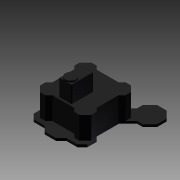
# Autodesk Inventor part: Base
Saved by Autodesk Inventor 2012 (Build 160160000, 160)
## iProperties
Created: 2013-03-08
Part Number: Base
Material: Default
Document SubType Name: Modeling
Designer: Andrew
Density: 1 g/cm^3
Author: Andrew
Autodesk Inventor part; units mm, degrees
ref_plane "YZ Plane" through (0, 0, 0) normal (1, 0, 0) x (0, 1, 0)
ref_plane "XZ Plane" through (0, 0, 0) normal (0, 1, 0) x (-1, 0, 0)
ref_plane "XY Plane" through (0, 0, 0) normal (0, 0, 1) x (1, 0, 0)
sketch "Sketch1" plane through (0, 0, 0) normal (0, 0, 1) x (1, 0, 0)
  line L0 (87.39809, 90.638849) -> (76.791489, 101.245451)
  line L1 (110.603697, 90.638591) -> (87.39809, 90.638849)
  line L2 (121.210063, 101.244956) -> (110.603697, 90.638591)
  line L3 (143.419374, 101.244709) -> (121.210063, 101.244956)
  line L4 (153.419263, 111.244598) -> (143.419374, 101.244709)
  line L5 (153.419473, 130.081843) -> (153.419263, 111.244598)
  line L6 (144.001258, 139.500058) -> (153.419473, 130.081843)
  line L7 (144.001258, 184.500058) -> (144.001258, 139.500058)
  line L8 (162.838724, 203.336883) -> (144.001258, 184.500058)
  line L9 (174.479779, 203.336684) -> (162.838724, 203.336883)
  line L10 (188.623093, 217.476415) -> (174.479779, 203.336684)
  line L11 (188.623904, 237.476415) -> (188.623093, 217.476415)
  line L12 (174.481567, 251.622561) -> (188.623904, 237.476415)
  line L13 (154.481567, 251.622902) -> (174.481567, 251.622561)
  line L14 (140.33919, 237.481007) -> (154.481567, 251.622902)
  line L15 (140.338992, 225.83779) -> (140.33919, 237.481007)
  line L16 (121.502223, 207.001664) -> (140.338992, 225.83779)
  line L17 (76.502223, 207.001664) -> (121.502223, 207.001664)
  line L18 (57.665842, 225.839164) -> (76.502223, 207.001664)
  line L19 (57.66604, 237.480627) -> (57.665842, 225.839164)
  line L20 (43.524145, 251.623004) -> (57.66604, 237.480627)
  line L21 (23.524145, 251.623344) -> (43.524145, 251.623004)
  line L22 (9.381769, 237.48145) -> (23.524145, 251.623344)
  line L23 (9.380958, 217.48145) -> (9.381769, 237.48145)
  line L24 (23.52252, 203.338741) -> (9.380958, 217.48145)
  line L25 (35.165328, 203.338269) -> (23.52252, 203.338741)
  line L26 (54.001421, 184.501058) -> (35.165328, 203.338269)
  line L27 (54.001421, 139.501058) -> (54.001421, 184.501058)
  line L28 (44.582671, 130.082867) -> (54.001421, 139.501058)
  line L29 (44.582461, 111.245809) -> (44.582671, 130.082867)
  line L30 (54.582226, 101.245698) -> (44.582461, 111.245809)
  line L31 (76.791489, 101.245451) -> (54.582226, 101.245698)
  circle A0 centre (99, 132) radius 5.5
  arc A1 (130.06, 142) -> (135.06, 142) centre (132.56, 142) ccw
  line L32 (130.06, 142) -> (130.06, 182)
  line L33 (135.06, 182) -> (135.06, 142)
  arc A2 (62.940969, 142) -> (67.940969, 142) centre (65.440969, 142) ccw
  arc A3 (67.940969, 182) -> (62.940969, 182) centre (65.440969, 182) ccw
  line L34 (67.940969, 182) -> (67.940969, 142)
  line L35 (138.997508, 214.221497) -> (150.997508, 202.221497)
  line L36 (128.721743, 214.221497) -> (138.997508, 214.221497)
  line L37 (121.5, 207) -> (128.721743, 214.221497)
  line L38 (76.5, 207) -> (121.5, 207)
  line L39 (69.278592, 214.221497) -> (76.5, 207)
  line L40 (59.002492, 214.221497) -> (69.278592, 214.221497)
  line L41 (47.002492, 202.221497) -> (59.002492, 214.221497)
  line L42 (47.002492, 191.497594) -> (47.002492, 202.221497)
  line L43 (54, 184.5) -> (47.002492, 191.497594)
  line L44 (54, 139.5) -> (54, 184.5)
  line L45 (47.002492, 132.502579) -> (54, 139.5)
  line L46 (47.002492, 121.778503) -> (47.002492, 132.502579)
  line L47 (59.002492, 109.778503) -> (47.002492, 121.778503)
  line L48 (69.278414, 109.778503) -> (59.002492, 109.778503)
  line L49 (76.5, 117) -> (69.278414, 109.778503)
  line L50 (121.5, 117) -> (76.5, 117)
  line L51 (128.721408, 109.778503) -> (121.5, 117)
  line L52 (138.997508, 109.778503) -> (128.721408, 109.778503)
  line L53 (150.997508, 121.778503) -> (138.997508, 109.778503)
  line L54 (150.997508, 132.502406) -> (150.997508, 121.778503)
  line L55 (144, 139.5) -> (150.997508, 132.502406)
  line L56 (144, 184.5) -> (144, 139.5)
  line L57 (150.997508, 191.497269) -> (144, 184.5)
  line L58 (150.997508, 202.221497) -> (150.997508, 191.497269)
  arc A4 (99.74629, 120.775345) -> (99.246799, 120.752769) centre (99, 131.75) ccw
  line L59 (111.585786, 133.75) -> (111, 133.75)
  line L60 (111.585786, 133.75) -> (111.585786, 135.25)
  line L61 (111.585786, 135.25) -> (113.5, 135.25)
  line L62 (113.5, 135.45) -> (113.5, 135.25)
  line L63 (113.5, 135.45) -> (113.917157, 135.45)
  line L64 (113.917157, 135.45) -> (113.917157, 141.55)
  line L65 (110.05, 169.167157) -> (103.95, 169.167157)
  line L66 (103.95, 169.167157) -> (103.95, 166.667157)
  line L67 (103.95, 166.667157) -> (94.05, 166.667157)
  line L68 (94.05, 166.667157) -> (94.05, 169.167157)
  line L69 (87.95, 169.167157) -> (87.95, 168.75)
  line L70 (87.95, 168.75) -> (87.5, 168.75)
  line L71 (86.414214, 135.25) -> (84.5, 135.25)
  line L72 (86.414214, 135.25) -> (86.414214, 133.75)
  line L73 (86.414214, 133.75) -> (87, 133.75)
  line L74 (87, 133.75) -> (87, 125.5)
  line L75 (87, 125.5) -> (89, 125.5)
  line L76 (109, 125.5) -> (111, 125.5)
  line L77 (111, 125.5) -> (111, 133.75)
  line L78 (85, 136.25) -> (86, 136.25)
  line L79 (86, 136.25) -> (86, 137.354356)
  line L80 (104.686492, 167.25) -> (104.686492, 168.25)
  line L81 (104.686492, 168.25) -> (105.854356, 168.25)
  line L82 (105.854356, 167.25) -> (104.686492, 167.25)
  circle A5 centre (99, 131.75) radius 11
  point P0 (0, 0)
  point P1 (0, 0)
  constraints: 64 end point, 1 centre point, 1 coincident, 1 concentric
extrude "Extrusion1" add sketch "Sketch1" along normal blind 5 contours L0 L31 L30 L29 L28 L46 L47 L48 L49 L50 L51 L52 L53 L54 L6 L5 L4 L3 L2 L1 | L28 L27 L26 L42 L41 L40 L39 L17 L16 L36 L35 L58 L8 L7 L6 L54 L53 L52 L51 L50 L49 L48 L47 L46 | L26 L25 L24 L23 L22 L21 L20 L19 L18 L39 L40 L41 L42 | L58 L35 L36 L16 L15 L14 L13 L12 L11 L10 L9 L8 | A0 | A5 A4
extrude "Extrusion2" add sketch "Sketch1" along normal blind 50.4 contours L28 L27 L26 L42 L41 L40 L39 L17 L16 L36 L35 L58 L8 L7 L6 L54 L53 L52 L51 L50 L49 L48 L47 L46 | A0 | A5 A4
extrude "Extrusion3" add sketch "Sketch1" along normal blind 87.4 contours A0 | A5 A4
sketch "Sketch2" plane through (0, 0, 50.4) normal (0, 0, 1) x (1, 0, 0)
  circle A0 centre (99, 131.75) radius 11 projected
  line L0 (144, 184.5) -> (144, 139.5) projected
  line L1 (99, 120.75) -> (112, 120.75)
  line L2 (112, 120.75) -> (112, 165.75)
  line L3 (112, 165.75) -> (86, 165.75)
  line L4 (86, 165.75) -> (86, 120.75)
  line L5 (86, 120.75) -> (99, 120.75)
  point P0 (0, 0)
  dimension "d6" = 13
  dimension "d7" = 45
  dimension "d8" = 26
  constraints: 10 end point, 2 parallel, 2 perpendicular, 1 horizontal, 1 vertical alignment, 1 other
  measures "d6" distance of L1.start L1.end
  measures "d7" distance of L1.end L2.end
  measures "d8" distance of L2.end L3.end
extrude "Extrusion4" add sketch "Sketch2" along normal blind 34
fillet "Fillet1" radius 2 7 edges at (112, 165.75, 67.4) (112, 143.25, 84.4) (112, 120.75, 67.4) (86, 120.75, 67.4) (86, 143.25, 84.4) (99, 165.75, 84.4) (86, 165.75, 67.4)
body "Solid1"
